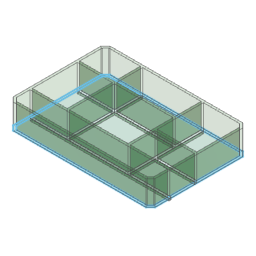
_Case Outline.a61dcd74-5b20-4951-86ae-bdb80058c364 (Autodesk Fusion 360 design; units mm, degrees)
Autodesk Fusion 360 part; units mm, degrees
sketch "Sketch1" plane through (0, 0, 0) normal (0, 0, 1) x (1, 0, 0)
  line L0 (-400.05, 260.35) -> (-387.35, 273.05)
  line L1 (-400.05, 12.7) -> (-387.35, 0)
  line L2 (-400.05, 260.35) -> (-400.05, 12.7)
  line L3 (0, 260.35) -> (-12.7, 273.05)
  line L4 (0, 12.7) -> (-12.7, 0)
  line L5 (0, 260.35) -> (0, 12.7)
  line L6 (-387.35, 0) -> (-12.7, 0)
  line L7 (-387.35, 273.05) -> (-12.7, 273.05)
  line L8 (-6.35, 257.7197) -> (-15.3303, 266.7)
  line L9 (-384.7197, 266.7) -> (-15.3303, 266.7)
  line L10 (-393.7, 257.7197) -> (-384.7197, 266.7)
  line L11 (-393.7, 257.7197) -> (-393.7, 15.3303)
  line L12 (-393.7, 15.3303) -> (-384.7197, 6.35)
  line L13 (-384.7197, 6.35) -> (-15.3303, 6.35)
  line L14 (-6.35, 15.3303) -> (-15.3303, 6.35)
  line L15 (-6.35, 257.7197) -> (-6.35, 15.3303)
  dimension "d5" = 6.35
  constraint vertical L2
  constraint horizontal L6
  constraint parallel L6 L7
extrude "Extrude1" add sketch "Sketch1" along normal blind 0.254 contours L0 L1 L2 L3 L4 L5 L6 L7 | L8 L9 L10 L11 L12 L13 L14 L15
extrude "Extrude2" add sketch "Sketch1" along normal blind 69.85
sketch "Sketch2" plane through (0, 0, 69.85) normal (0, 0, 1) x (-1, 0, 0)
  line L0 (393.7, -15.3303) -> (393.7, -257.7197)
  line L1 (393.7, -257.7197) -> (384.7197, -266.7)
  line L2 (384.7197, -266.7) -> (15.3303, -266.7)
  line L3 (15.3303, -266.7) -> (6.35, -257.7197)
  line L4 (6.35, -257.7197) -> (6.35, -15.3303)
  line L5 (6.35, -15.3303) -> (15.3303, -6.35)
  line L6 (15.3303, -6.35) -> (384.7197, -6.35)
  line L7 (384.7197, -6.35) -> (393.7, -15.3303)
  line L8 (400.05, -260.35) -> (400.05, -12.7)
  line L9 (400.05, -12.7) -> (387.35, 0)
  line L10 (387.35, 0) -> (12.7, 0)
  line L11 (12.7, 0) -> (0, -12.7)
  line L12 (0, -12.7) -> (0, -260.35)
  line L13 (0, -260.35) -> (12.7, -273.05)
  line L14 (12.7, -273.05) -> (387.35, -273.05)
  line L15 (387.35, -273.05) -> (400.05, -260.35)
  line L16 (393.7, -162.4342) -> (393.7, -166.61)
  line L17 (295.275, -266.7) -> (288.925, -266.7)
  line L18 (393.7, -193.675) -> (295.275, -193.675)
  line L19 (393.7, -193.675) -> (295.275, -193.675)
  line L20 (295.275, -193.675) -> (295.275, -187.325)
  line L21 (295.275, -187.325) -> (393.7, -187.325)
  line L22 (393.7, -187.325) -> (393.7, -193.675)
  line L23 (295.275, -187.325) -> (295.275, -193.675)
  line L24 (2.1633, -60.325) -> (288.925, -60.325)
  line L25 (288.925, -60.325) -> (288.925, -187.325)
  line L26 (2.1633, -60.325) -> (393.7, -60.325)
  line L27 (393.7, -60.325) -> (393.7, -53.975)
  line L28 (393.7, -53.975) -> (2.1633, -53.975)
  line L29 (2.1633, -53.975) -> (2.1633, -60.325)
  line L30 (295.275, -53.975) -> (288.925, -53.975)
  line L31 (288.925, -187.325) -> (123.825, -187.325)
  line L32 (123.825, -187.325) -> (117.475, -187.325)
  line L33 (117.475, -187.325) -> (123.825, -187.325)
  line L34 (123.825, -187.325) -> (123.825, -60.325)
  line L35 (123.825, -60.325) -> (117.475, -60.325)
  line L36 (117.475, -60.325) -> (117.475, -187.325)
  line L37 (295.275, -187.325) -> (288.925, -187.325)
  line L38 (288.925, -187.325) -> (288.925, -60.325)
  line L39 (288.925, -60.325) -> (295.275, -60.325)
  line L40 (295.275, -60.325) -> (295.275, -187.325)
  line L41 (295.275, -266.7) -> (288.925, -266.7)
  line L42 (288.925, -266.7) -> (288.925, -193.675)
  line L43 (288.925, -193.675) -> (295.275, -193.675)
  line L44 (295.275, -193.675) -> (295.275, -266.7)
  line L45 (117.475, -60.325) -> (123.825, -60.325)
  line L46 (123.825, -60.325) -> (123.825, -130.175)
  line L47 (123.825, -130.175) -> (117.475, -130.175)
  line L48 (117.475, -130.175) -> (117.475, -60.325)
  line L49 (117.475, -130.175) -> (6.35, -130.175)
  line L50 (6.35, -130.175) -> (6.35, -136.525)
  line L51 (6.35, -136.525) -> (117.475, -136.525)
  line L52 (117.475, -136.525) -> (117.475, -130.175)
  line L53 (117.475, -187.325) -> (393.7, -187.325)
  line L54 (393.7, -187.325) -> (393.7, -193.675)
  line L55 (393.7, -193.675) -> (117.475, -193.675)
  line L56 (117.475, -193.675) -> (117.475, -187.325)
  line L57 (123.825, -193.675) -> (117.475, -193.675)
  line L58 (117.475, -193.675) -> (117.475, -266.7)
  line L59 (117.475, -266.7) -> (123.825, -266.7)
  line L60 (123.825, -266.7) -> (123.825, -193.675)
  dimension "d11" = 6.35
  dimension "d12" = 73.025
  dimension "d13" = 6.35
  dimension "d15" = 6.35
  dimension "d17" = 6.35
  dimension "d18" = 165.1
  dimension "d19" = 6.35
  dimension "d22" = 127
  dimension "d23" = 6.35
  dimension "d24" = 69.85
  dimension "d25" = 6.35
  constraint vertical L16
  constraint coincident L0 L16.end
  constraint horizontal L17
  constraint coincident L2 L17.start
  constraint horizontal L18
  constraint horizontal L19
  constraint vertical L20
  constraint horizontal L21
  constraint vertical L22
  constraint vertical L23
  constraint horizontal L24
  constraint vertical L25
  constraint horizontal L26
  constraint vertical L27
  constraint horizontal L28
  constraint vertical L29
  constraint horizontal L30
  constraint coincident L28 L30.start
  constraint horizontal L31
  constraint horizontal L32
  constraint horizontal L33
  constraint vertical L34
  constraint horizontal L35
  constraint vertical L36
  constraint horizontal L37
  constraint vertical L38
  constraint horizontal L39
  constraint vertical L40
  constraint horizontal L41
  constraint vertical L42
  constraint horizontal L43
  constraint vertical L44
  constraint horizontal L45
  constraint vertical L46
  constraint horizontal L47
  constraint vertical L48
  constraint horizontal L49
  constraint vertical L50
  constraint horizontal L51
  constraint vertical L52
  constraint coincident L4 L50.end
  constraint horizontal L53
  constraint vertical L54
  constraint horizontal L55
  constraint vertical L56
  constraint horizontal L57
  constraint vertical L58
  constraint horizontal L59
  constraint vertical L60
  constraint coincident L2 L58.end
  constraint coincident L55 L57.start
  measures "d11" distance of L17.start L17.end
  measures "d12" distance of L17.start L18.end
  measures "d13" distance of L18.start L21.end
  measures "d15" distance of L18.end L20.end
  measures "d17" distance of L24.start L28.end
  measures "d18" distance of L25.end L31.end
  measures "d19" distance of L31.end L32.end
  measures "d22" distance of L25.end L24.end
  measures "d23" distance of L32.end L31.end
  measures "d24" distance of L35.end L47.end
  measures "d25" distance of L47.end L51.end
extrude "Extrude3" add sketch "Sketch2" against normal blind 76.2 contours L0 L4 L24 L26 L27 L28 L30 L35 L39 L45 | L25 L26 L37 L38 L39 L40 L53 | L0 L18 L19 L20 L21 L22 L23 L53 L54 L55 | L20 L23 L31 L32 L33 L37 L43 L53 L55 L56 L57 | L4 L24 L26 L28 L29 | L24 L26 L34 L35 L36 L45 L46 L47 L48 | L2 L17 L41 L42 L43 L44 L55 | L32 L33 L34 L36 L47 L52 L53 | L4 L36 L49 L50 L51 L52 | L2 L55 L57 L58 L59 L60
